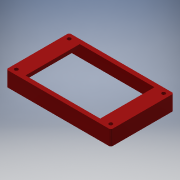
# Autodesk Inventor part: front_case
Saved by Autodesk Inventor 2018.2 (Build 222227000, 227)
## iProperties
Created: 2018-04-02
Part Number: front_case
Material: ABS-Kunststoff
Document SubType Name: Modeling
Designer: Till
Density: 1.06 g/cm^3
Appearance: Rot
Author: Till
Autodesk Inventor part; units mm, degrees
ref_plane "YZ Plane" through (0, 0, 0) normal (1, 0, 0) x (0, 1, 0)
ref_plane "XZ Plane" through (0, 0, 0) normal (0, 1, 0) x (-1, 0, 0)
sketch "Skizze1" plane through (0, 0, 0) normal (0, 0, 1) x (1, 0, 0)
  line L0 (-40.3, -29.3) -> (40.3, -29.3)
  line L1 (40.3, -29.3) -> (40.3, 29.3)
  line L2 (40.3, 29.3) -> (-40.3, 29.3)
  line L3 (-40.3, 29.3) -> (-40.3, -29.3)
  line L4 (40, 29) -> (-40, 29) projected
  line L5 (-40, 29) -> (-40, -29) projected
  line L6 (-40, -29) -> (40, -29) projected
  line L7 (40, -29) -> (40, 29) projected
  line L8 (-56.5, -34) -> (56.5, -34)
  line L9 (56.5, -34) -> (56.5, 34)
  line L10 (56.5, 34) -> (-56.5, 34)
  line L11 (-56.5, 34) -> (-56.5, -34)
  line L12 (53, 32.5) -> (-53, 32.5) projected
  line L13 (-53, -32.5) -> (53, -32.5) projected
  line L14 (55, -30.5) -> (55, 30.5) projected
  line L15 (-55, 30.5) -> (-55, -30.5) projected
  circle A0 centre (-51, 28.5) radius 2 projected
  circle A1 centre (51, 28.5) radius 2 projected
  circle A2 centre (51, -28.5) radius 2 projected
  circle A3 centre (-51, -28.5) radius 2 projected
  point P0 (0, 0)
  dimension "d0" = 0.3
  dimension "d1" = 0.3
  dimension "d2" = 0.3
  dimension "d3" = 0.3
  dimension "d4" = 1.5
  dimension "d5" = 1.5
  dimension "d6" = 1.5
  dimension "d7" = 1.5
  constraints: 16 end point, 4 parallel, 2 horizontal, 2 perpendicular
  measures "d0" distance between parallel lines of L2 L4
  measures "d1" distance between parallel lines of L7 L1
  measures "d2" distance between parallel lines of L6 L0
  measures "d3" distance between parallel lines of L5 L3
  measures "d4" distance between parallel lines of L10 L12
  measures "d5" distance between parallel lines of L15 L11
  measures "d6" distance between parallel lines of L8 L13
  measures "d7" distance between parallel lines of L9 L14
extrude "Extrusion1" add sketch "Skizze1" against normal blind 1.2 contours L11 L10 L9 L8
sketch "Skizze2" plane through (0, 0, -1.2) normal (0, 0, -1) x (-1, 0, 0)
  circle A0 centre (-51, 28.5) radius 2 projected
  circle A1 centre (51, 28.5) radius 2 projected
  circle A2 centre (51, -28.5) radius 2 projected
  circle A3 centre (-51, -28.5) radius 2 projected
  circle A4 centre (-51, 28.5) radius 3
  circle A5 centre (51, 28.5) radius 3
  circle A6 centre (-51, -28.5) radius 3
  circle A7 centre (51, -28.5) radius 3
  line L0 (-40.3, -29.3) -> (-40.3, 29.3) projected
  line L1 (-40.3, 29.3) -> (40.3, 29.3) projected
  line L2 (-40.3, -29.3) -> (40.3, -29.3)
  line L3 (40.3, -29.3) -> (40.3, 29.3)
  line L4 (40.3, 29.3) -> (-40.3, 29.3)
  line L5 (-40.3, 29.3) -> (-40.3, -29.3)
  line L6 (41.5, 30.5) -> (-41.5, 30.5)
  line L7 (-41.5, 30.5) -> (-41.5, -30.5)
  line L8 (-41.5, -30.5) -> (41.5, -30.5)
  line L9 (41.5, -30.5) -> (41.5, 30.5)
  point P0 (0, 0)
  point P1 (53.2361, -26.5)
  point P2 (48.7639, -26.5)
  point P3 (51, -26.5)
  dimension "d10" = 6
  dimension "d11" = 6
  dimension "d12" = 6
  dimension "d13" = 6
  dimension "d14" = 1.2
  dimension "d15" = 1.2
  dimension "d16" = 1.2
  dimension "d17" = 1.2
  constraints: 16 end point, 4 centre point, 4 coincident, 4 parallel, 2 horizontal, 2 perpendicular, 2 point on circle, 1 vertical alignment, 1 other
  measures "d10" diameter of A4
  measures "d11" diameter of A5
  measures "d12" diameter of A6
  measures "d13" diameter of A7
  measures "d14" distance between parallel lines of L1 L6
  measures "d15" distance between parallel lines of L5 L7
  measures "d16" distance between parallel lines of L3 L9
  measures "d17" distance between parallel lines of L2 L8
ref_plane "Arbeitsebene1" through (-55, -32.5, -4) normal (0, 0, 1) x (1, 0, 0)
extrude "Extrusion2" add sketch "Skizze2" along normal up to surface (2.8 mm away)
sketch "Skizze3" plane through (0, 0, -1.2) normal (0, 0, -1) x (-1, 0, 0)
  line L0 (-56.5, -34) -> (56.5, -34) projected
  line L1 (-56.5, 34) -> (-56.5, -34) projected
  line L2 (56.5, -34) -> (-56.5, -34)
  line L3 (-56.5, -34) -> (-56.5, 34)
  line L4 (-56.5, 34) -> (56.5, 34)
  line L5 (56.5, 34) -> (56.5, -34)
  line L6 (-55.3, 32.8) -> (55.3, 32.8)
  line L7 (55.3, 32.8) -> (55.3, -32.8)
  line L8 (55.3, -32.8) -> (-55.3, -32.8)
  line L9 (-55.3, -32.8) -> (-55.3, 32.8)
  point P0 (0, 0)
  dimension "d20" = 1.2
  dimension "d21" = 1.2
  dimension "d22" = 1.2
  dimension "d23" = 1.2
  constraints: 16 end point, 4 parallel, 2 horizontal, 2 perpendicular
  measures "d20" distance between parallel lines of L5 L7
  measures "d21" distance between parallel lines of L0 L8
  measures "d22" distance between parallel lines of L1 L9
  measures "d23" distance between parallel lines of L4 L6
extrude "Extrusion3" add sketch "Skizze3" along normal blind 15
fillet "Rundung1" radius 2 8 edges at (55.3, 32.8, -8.7) (-55.3, 32.8, -8.7) (-55.3, -32.8, -8.7) (56.5, -34, -8.1) (-56.5, -34, -8.1) (-56.5, 34, -8.1) (56.5, 34, -8.1) (55.3, -32.8, -8.7)
sketch "Skizze4" plane through (-56.5, -32, 0) normal (-1, 0, 0) x (0, 0, 1)
  line L0 (-5.5, 1.5) -> (-5.5, 5.5) construction
  line L1 (-5.5, 1.5) -> (-4, 1.5) construction
  line L2 (-4, 62.5) -> (-4, 1.5) construction
  line L3 (-5.5, 62.5) -> (-4, 62.5) construction
  line L4 (-5.5, 56.5) -> (-5.5, 62.5) construction
  line L5 (-5.5, 56.5) -> (-8.3, 56.5) construction
  line L6 (-8.3, 26.5) -> (-8.3, 56.5) construction
  line L7 (-5.5, 26.5) -> (-8.3, 26.5) construction
  line L8 (-5.5, 20) -> (-5.5, 26.5) construction
  line L9 (-5.5, 20) -> (-13.5, 20) construction
  line L10 (-13.5, 5.5) -> (-13.5, 20) construction
  line L11 (-5.5, 5.5) -> (-13.5, 5.5) construction
  line L12 (-5, 20.5) -> (-14, 20.5)
  line L13 (-14, 20.5) -> (-14, 5)
  line L14 (-14, 5) -> (-5, 5)
  line L15 (-5, 5) -> (-5, 20.5)
  line L16 (-5, 26) -> (-8.8, 26)
  line L17 (-8.8, 26) -> (-8.8, 57)
  line L18 (-8.8, 57) -> (-5, 57)
  line L19 (-5, 57) -> (-5, 26)
  point P0 (0, 32)
  dimension "d27" = 0.5
  dimension "d28" = 0.5
  dimension "d29" = 0.5
  dimension "d30" = 0.5
  dimension "d31" = 0.5
  dimension "d32" = 0.5
  dimension "d33" = 0.5
  constraints: 16 end point, 4 parallel, 2 horizontal, 2 perpendicular, 1 point on line
  measures "d27" distance between parallel lines of L13 L10
  measures "d28" distance between parallel lines of L11 L14
  measures "d29" distance between parallel lines of L12 L9
  measures "d30" distance between parallel lines of L8 L15
  measures "d31" distance between parallel lines of L7 L16
  measures "d32" distance between parallel lines of L6 L17
  measures "d33" distance between parallel lines of L18 L5
extrude "Extrusion4" cut sketch "Skizze4" against normal up to next
